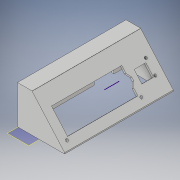
# Autodesk Inventor part: Suport - pantalla i potenciometre
Saved by Autodesk Inventor 2019 (Build 230136000, 136)
## iProperties
Created: 2018-08-18
Part Number: Suport - pantalla i potenciometre
Material: Genérico
Document SubType Name: Modeling
Designer: Albert Garangou Culebras
Density: 1 g/cm^3
Appearance: Valor por defecto
Author: Albert Garangou Culebras
Autodesk Inventor part; units mm, degrees
ref_plane "YZ Plane" through (0, 0, 0) normal (1, 0, 0) x (0, 1, 0)
ref_plane "XZ Plane" through (0, 0, 0) normal (0, 1, 0) x (-1, 0, 0)
ref_plane "XY Plane" through (0, 0, 0) normal (0, 0, 1) x (1, 0, 0)
sketch "Boceto3" plane through (0, 0, 0) normal (0, 0, 1) x (1, 0, 0)
  line L0 (40, 0) -> (37, 0)
  line L1 (0, 0) -> (0, 45)
  line L2 (0, 45) -> (3, 45)
  line L3 (40, 0) -> (40, 3)
  line L4 (40, 3) -> (3, 45)
  line L5 (0, 0) -> (40, 0)
  dimension "d3" = 3
  dimension "d4" = 45
  dimension "d5" = 3
  dimension "d6" = 3
  constraints: 12 end point, 2 horizontal, 2 vertical, 1 perpendicular
  measures "d3" distance of L0.start L0.end
  measures "d4" distance of L1.start L1.end
  measures "d5" distance of L1.end L2.end
  measures "d6" distance of L0.start L3.end
extrude "Extrusión1" add sketch "Boceto3" against normal blind 98.2
sketch "Boceto4" plane through (0, 0, 0) normal (0, 0, 1) x (1, 0, 0)
  line L0 (3.3154, 41.6201) -> (2, 43)
  line L1 (3.3154, 41.6201) -> (38, 2)
  line L2 (38, 2) -> (2, 2)
  line L3 (2, 2) -> (2, 43)
  point P0 (0, 45)
  constraints: 8 end point, 1 horizontal
extrude "Extrusión2" cut sketch "Boceto4" against normal blind 210.55
sketch "Boceto6" plane through (0, 0, 0) normal (0, 0, 1) x (1, 0, 0)
  line L0 (1.0395, 0.9992) -> (39.0395, 0.9992)
  line L1 (39.0395, 1.0003) -> (39.0395, 1.9993) projected
  line L2 (39.0395, 0.9992) -> (39.0395, 1.9993)
  line L3 (39.0395, 1.9993) -> (3, 44.0003)
  line L4 (2.88, 44.0003) -> (1, 44.0003) projected
  line L5 (3, 44.0003) -> (1, 44.0003)
  line L6 (1, 1.0003) -> (39.0395, 1.0003) projected
  line L7 (1, 44.0003) -> (1, 1.0003)
  point P0 (0, 0)
  constraints: 10 end point, 2 perpendicular, 1 horizontal, 1 parallel
extrude "Extrusión3" add sketch "Boceto6" against normal blind 2
sketch "Boceto7" plane through (0, 0, -98.2) normal (0, 0, -1) x (-1, 0, 0)
  line L0 (-1, 1.0003) -> (-39.0395, 1.0003) projected
  line L1 (-1, 1.0003) -> (-39.0395, 1.0003)
  line L2 (-39.0395, 1.0003) -> (-39.0395, 2)
  line L3 (-39.0395, 1.9993) -> (-2.88, 44.0003) projected
  line L4 (-39.0395, 2) -> (-2.88, 44.0003)
  line L5 (-2.88, 44.0003) -> (-1, 44.0003) projected
  line L6 (-1, 44.0003) -> (-1, 1.0003)
  line L7 (-2.88, 44.0003) -> (6.9067, 55.3678)
  line L8 (6.9067, 55.3678) -> (10.1689, 59.157)
  line L9 (10.1689, 59.157) -> (10.1689, 0)
  line L10 (10.1689, 0) -> (0, 0)
  dimension "d68" = 15
  dimension "d70" = 5
  constraints: 17 end point, 2 perpendicular, 2 vertical, 1 collinear
  measures "d68" distance of L3.end L7.end
  measures "d70" distance of L7.end L8.end
extrude "Extrusión4" add sketch "Boceto7" against normal blind 2
sketch "Boceto10" plane through (0, 0, -96.2) normal (0, 0, 1) x (1, 0, 0)
  line L0 (20.1691, 1.0003) -> (21.6691, 1.0003)
  line L1 (39.0395, 1.0003) -> (1, 1.0003) projected
  line L2 (21.6691, 1.0003) -> (21.6691, 22.1759)
  line L3 (2.88, 44.0003) -> (39.0395, 1.9993) projected
  line L4 (21.6691, 22.1759) -> (20.1691, 23.9182)
  line L5 (20.1691, 23.9182) -> (20.1691, 1.0003)
  point P0 (0, 0)
  dimension "d49" = 1.5
  constraints: 8 end point, 2 point on line, 1 collinear, 1 parallel, 1 vertical
  measures "d49" distance of L0.start L0.end
extrude "Extrusión7" add sketch "Boceto10" along normal blind 96
sketch "Boceto15" plane through (0, 0, -98.2) normal (0, 0, -1) x (-1, 0, 0)
  line L0 (-3, 45) -> (-40, 3) projected
  line L1 (-20.3927, 25.257) -> (-7.1721, 40.2641)
  line L2 (-7.1721, 40.2641) -> (-7.1721, 0)
  line L3 (-20.1691, 1.0003) -> (-1, 1.0003) projected
  line L4 (-7.1721, 40.2641) -> (-3, 45)
  line L5 (0, 45) -> (-3, 45)
  line L6 (0, 0) -> (0, 45) projected
  line L7 (0, 45) -> (0, 0)
  line L8 (0, 0) -> (-7.1721, 0)
  line L9 (-40, 0) -> (0, 0) projected
  dimension "d71" = 20
  constraints: 12 end point, 3 collinear, 2 point on line, 1 horizontal, 1 perpendicular
  measures "d71" distance of L1.start L1.end
extrude "Extrusión9" cut sketch "Boceto15" against normal blind 617.4
sketch "Boceto16" plane through (0, 0, -96.2) normal (0, 0, 1) x (1, 0, 0)
  line L0 (7.1721, 1) -> (8.6721, 1.0003)
  line L1 (20.1691, 1.0003) -> (7.1721, 1.0003) projected
  line L2 (8.6721, 1.0003) -> (8.6721, 37.2725)
  line L3 (7.1721, 39.0149) -> (20.1691, 23.9182) projected
  line L4 (8.6721, 37.2725) -> (7.1721, 39.0149)
  line L5 (7.1721, 39.0149) -> (7.1721, 1)
  point P0 (0, 0)
  dimension "d74" = 1.5
  constraints: 8 end point, 1 collinear, 1 parallel, 1 perpendicular, 1 point on line
  measures "d74" distance of L0.start L0.end
extrude "Extrusión10" add sketch "Boceto16" along normal blind 95.4
sketch "Boceto17" plane through (0, 0, 0) normal (0, 0, 1) x (1, 0, 0)
  line L0 (20.1691, 1.0003) -> (8.6721, 1.0003) projected
  line L1 (8.6721, 35.5011) -> (8.6721, 2) projected
  line L2 (8.6721, 1.0003) -> (8.6721, 37.2725)
  line L3 (39.0395, 1.9993) -> (21.6691, 22.1759) projected
  line L4 (8.6721, 37.2725) -> (39.0395, 1.9993)
  line L5 (39.0395, 1.9993) -> (39.0395, 1.0003)
  line L6 (39.0395, 1.0003) -> (8.6721, 1.0003)
  line L7 (40, 0) -> (7.1721, 0) projected
  point P0 (0, 0)
  constraints: 8 end point, 2 collinear, 2 parallel
extrude "Extrusión11" cut sketch "Boceto17" against normal blind 235.6
sketch "Boceto21" plane through (40, 3, 0) normal (0.750359, 0.6610305, 0) x (0, 0, -1)
  line L0 (85, 24.1901) -> (85, 18.1901)
  line L1 (76, 24.1901) -> (81, 24.1901)
  line L2 (81, 24.1901) -> (85, 24.1901)
  line L3 (77, 12.1901) -> (76, 12.1901)
  line L4 (77, 12.1901) -> (77, 11.1901)
  line L5 (5, 11.1901) -> (5, 12.1901)
  line L6 (5, 11.1901) -> (5, 7.1901)
  line L7 (5, 7.1901) -> (77, 7.1901)
  line L8 (77, 7.1901) -> (77, 11.1901)
  line L9 (77, 32.1901) -> (5, 32.1901)
  line L10 (5, 7.1901) -> (5, 32.1901)
  line L11 (77, 12.1901) -> (77, 32.1901)
  line L12 (85, 18.1901) -> (85, 13.1901)
  line L13 (98.2, 19.2082) -> (98.2, -0.8655) projected
  line L14 (97, 18.1901) -> (97, 13.1901)
  line L15 (85, 13.1901) -> (97, 13.1901)
  line L16 (85, 25.1901) -> (97, 25.1901)
  line L17 (85, 24.1901) -> (85, 25.1901)
  line L18 (97, 25.1901) -> (97, 18.1901)
  line L19 (0, 19.2082) -> (98.2, 19.2082) projected
  point P0 (0, 24.1901)
  dimension "d114" = 5
  dimension "d177" = 1
  dimension "d184" = 4
  dimension "d186" = 5
  constraints: 36 end point, 4 vertical, 3 horizontal, 2 perpendicular, 1 point on line
  measures "d114" distance of L1.end L1.start
  measures "d177" distance of L3.start L4.end
  measures "d184" distance of L5.start L6.end
  measures "d186" distance of L0.end L12.end
extrude "Extrusión13" cut sketch "Boceto21" against normal blind 1.5 contours L17 L16 L18 L19 L0 | L19 L18 L14 L15 L12 L0 | L19 L10 L9 L11 | L11 L4 L8 L7 L6 L5 L10 L19
sketch "Boceto22" plane through (0, 0, 0) normal (0, 0, 1) x (1, 0, 0)
  line L0 (8.6721, 1.0003) -> (39.0395, 1.0003) projected
  line L1 (8.6721, 1.0003) -> (39.0395, 1.0003)
  line L2 (39.0395, 1.0003) -> (39.0395, 2)
  line L3 (39.0395, 2) -> (8.6721, 37)
  line L4 (8.6721, 37.2725) -> (8.6721, 1.0003) projected
  line L5 (8.6721, 37) -> (8.6721, 1.0003)
  line L6 (7.1721, 0) -> (7.1721, 40.2641) projected
  line L7 (7.1721, 40.2641) -> (7.1721, 0)
  line L8 (40, 3) -> (40, 0) projected
  line L9 (7.1721, 0) -> (40, 0)
  line L10 (40, 0) -> (40, 3)
  line L11 (40, 3) -> (7.1721, 40.2641)
  line L12 (7.1721, 40.2641) -> (40, 3) projected
  point P0 (0, 0)
  constraints: 16 end point, 3 collinear, 3 perpendicular, 1 horizontal
extrude "Extrusión14" add sketch "Boceto22" along normal blind 2
sketch "Boceto24" plane through (0, 0, 2) normal (0, 0, 1) x (1, 0, 0)
  line L0 (8.6721, 1.0003) -> (8.6721, 37) projected
  line L1 (39.0395, 1.0003) -> (8.6721, 1.0003) projected
  line L2 (8.6721, 1.0003) -> (39.0395, 1.0003)
  line L3 (39.0395, 1.0003) -> (39.0395, 2)
  line L4 (39.0395, 2) -> (8.6721, 37)
  line L5 (8.6721, 37) -> (8.6721, 1.0003)
  point P0 (0, 0)
  constraints: 8 end point, 1 collinear, 1 parallel, 1 perpendicular
extrude "Extrusión15" add sketch "Boceto24" against normal blind 2
sketch "Boceto25" plane through (0, 0, -98.2) normal (0, 0, -1) x (-1, 0, 0)
  line L0 (-8.6721, 1.0003) -> (-8.6721, 37.2725) projected
  line L1 (-8.6721, 1.0003) -> (-8.6721, 37.2725)
  line L2 (-8.6721, 37.2725) -> (-39, 2)
  line L3 (-39, 2) -> (-39, 1.0003)
  line L4 (-39, 1.0003) -> (-8.6721, 1.0003)
  line L5 (-7.1721, 0) -> (-40, 0) projected
  line L6 (-7.1721, 40) -> (-7.1721, 0)
  line L7 (-40, 0) -> (-7.1721, 0)
  line L8 (-40, 0) -> (-40, 2.8598)
  line L9 (-7.1721, 0) -> (-7.1721, 40.2641) projected
  line L10 (-40, 2.8598) -> (-7.1721, 40.2641)
  point P0 (0, 0)
  constraints: 16 end point, 2 parallel, 2 vertical, 1 collinear, 1 perpendicular
extrude "Extrusión16" add sketch "Boceto25" along normal blind 7
sketch "Boceto27" plane through (0, 0, -105.2) normal (0, 0, -1) x (-1, 0, 0)
  line L0 (-8.6721, 1.0003) -> (-39.0395, 1.0003) projected
  line L1 (-8.6721, 1.0003) -> (-39.0395, 1.0003)
  line L2 (-39.0395, 1.0003) -> (-39.0395, 1.9993)
  line L3 (-8.6721, 1.0003) -> (-8.6721, 37.2725) projected
  line L4 (-39.0395, 1.9993) -> (-8.6721, 37.2725)
  line L5 (-8.6721, 37.2725) -> (-8.6721, 1.0003)
  point P0 (0, 0)
  constraints: 8 end point, 2 collinear, 1 perpendicular
extrude "Extrusión17" add sketch "Boceto27" against normal blind 2
sketch "Boceto28" plane through (7.1721, 0, 2) normal (0, -1, 0) x (1, 0, 0)
  line L0 (0, 0) -> (0, -107.2) projected
  line L1 (32.8279, 0) -> (32.8279, -107.2) projected
  line L2 (0, 0) -> (32.8279, 0)
  line L3 (32.8279, 0) -> (32.8279, -107.2)
  line L4 (32.8279, -107.2) -> (0, -107.2)
  line L5 (0, -107.2) -> (0, 0)
  point P0 (-7.1721, -2)
  constraints: 8 end point, 2 parallel, 1 horizontal, 1 perpendicular
extrude "Extrusión18" add sketch "Boceto28" along normal blind 2
sketch "Boceto29" plane through (7.1721, 40.2641, -98.2) normal (-1, 0, 0) x (0, 0, 1)
  line L0 (0, 0) -> (-7, 0) projected
  line L1 (100.2, -37.2641) -> (100.2, -42.2641) projected
  line L2 (-7, 0) -> (100.2, 0)
  line L3 (100.2, 0) -> (100.2, -42.2641)
  line L4 (100.2, -42.2641) -> (-7, -42.2641)
  line L5 (-7, -42.2641) -> (-7, 0)
  point P0 (98.2, -40.2641)
  constraints: 8 end point, 2 parallel, 1 horizontal, 1 perpendicular
extrude "Extrusión19" add sketch "Boceto29" along normal blind 2
sketch "Boceto30" plane through (0, 0, -105.2) normal (0, 0, -1) x (-1, 0, 0)
  line L0 (-7.1721, 40.2641) -> (-5.1721, 40.2641)
  line L1 (-5.1721, 40.2641) -> (-5.1721, -2) projected
  line L2 (-5.1721, 40.2641) -> (-5.1721, -2)
  line L3 (-40, -2) -> (-5.1721, -2) projected
  line L4 (-5.1721, -2) -> (-40, -2)
  line L5 (-40, 2.8598) -> (-40, -2) projected
  line L6 (-40, -2) -> (-40, 2.8598)
  line L7 (-40, 2.8598) -> (-7.1721, 40.2641)
  line L8 (-7.1721, 40.2641) -> (-5.1721, 40.2641)
  point P0 (0, 0)
  constraints: 12 end point, 3 collinear, 1 horizontal, 1 perpendicular
extrude "Extrusión20" add sketch "Boceto30" along normal blind 2
sketch "Boceto31" plane through (0, 0, 2) normal (0, 0, 1) x (1, 0, 0)
  line L0 (5.1721, -2) -> (5.1721, 40.2641) projected
  line L1 (5.1721, 40.2643) -> (5.1721, -2)
  line L2 (40, -2) -> (5.1721, -2) projected
  line L3 (5.1721, -2) -> (40, -2)
  line L4 (40, 2.8598) -> (40, -2) projected
  line L5 (40, -2) -> (40, 2.8598)
  line L6 (40, 2.8598) -> (7.1721, 40.2641) projected
  line L7 (7.1721, 40.2641) -> (40, 2.8598)
  line L8 (7.1721, 40.2641) -> (5.1721, 40.2641)
  point P0 (0, 0)
  constraints: 11 end point, 3 collinear, 1 horizontal
extrude "Extrusión21" add sketch "Boceto31" along normal blind 2
sketch "Boceto32" plane through (40, 3, 2) normal (0.750359, 0.6610305, 0) x (0, 0, -1)
  line L0 (-2, 49.6617) -> (-2, 0)
  line L1 (-2, 0) -> (109.2, 0)
  line L2 (109.2, -3.7518) -> (109.2, 19.2705) projected
  line L3 (100.2, -0.1052) -> (109.2, -0.1052) projected
  line L4 (109.2, 49.6617) -> (109.2, -0.1052)
  line L5 (109.2, 49.6617) -> (-2, 49.6617)
  line L6 (-2, 50.9838) -> (-2, 19.2705) projected
  line L7 (7, 11.1901) -> (7, 36.1901) projected
  line L8 (7, 36.1901) -> (7, 12.1901)
  line L9 (78, 36.1901) -> (7, 36.1901)
  line L10 (87, 13.1901) -> (87, 25.1901) projected
  line L11 (100.2, 49.6617) -> (109.2, 49.6617) projected
  line L12 (109.2, 49.6617) -> (109.2, -0.1052)
  line L13 (-2, -3.7518) -> (-2, -0.1052) projected
  line L14 (109.2, -0.1052) -> (-2, -0.1052)
  line L15 (-2, -0.1052) -> (-2, 49.6617)
  line L16 (109.2, 49.6617) -> (-2, 49.6617)
  line L17 (7, 12.1901) -> (7, 11.1901)
  line L18 (7, 11.1901) -> (79, 11.1901)
  line L19 (79, 11.1901) -> (79, 36.1901)
  line L20 (79, 36.1901) -> (78, 36.1901)
  line L21 (99, 13.1901) -> (87, 13.1901) projected
  line L22 (99, 13.1901) -> (87, 13.1901)
  line L23 (87, 13.1901) -> (87, 25.1901)
  line L24 (99, 25.1901) -> (87, 25.1901) projected
  line L25 (99, 25.1901) -> (87, 25.1901)
  line L26 (99, 25.1901) -> (99, 13.1901)
  line L27 (100.2, 46.4254) -> (100.2, -0.0893) projected
  point P0 (2, 24.1901)
  point P1 (87, 30.1901)
  point P2 (99, 30.1901)
  point P3 (87, 18.1901)
  point P4 (99, 18.1901)
  dimension "d174" = 1
  dimension "d175" = 72
  constraints: 36 end point, 6 collinear, 5 perpendicular, 2 point on line, 2 vertical, 1 horizontal, 1 parallel
  measures "d174" distance of L8.end L7.start
  measures "d175" distance of L7.start L18.end
extrude "Extrusión22" [suppressed]
sketch "Boceto33" plane through (40.7504, 3.661, 2) normal (0.750359, 0.6610305, 0) x (0, 0, -1)
  line L0 (87, 25.1901) -> (87, 13.1901) projected
  line L1 (87, 30.1901) -> (99, 30.1901) projected
  line L2 (87, 30.1901) -> (99, 30.1901)
  line L3 (99, 30.1901) -> (99, 18.1338)
  line L4 (100.2, -0.1052) -> (100.2, 49.6617) projected
  line L5 (99, 18.1338) -> (87, 18.1338)
  line L6 (87, 30.1901) -> (87, 34.1901)
  line L7 (87, 34.1901) -> (83, 34.1901)
  line L8 (99, 18.1901) -> (99, 14.1901)
  line L9 (99, 14.1901) -> (103, 14.1901)
  line L10 (83, 34.1901) -> (103, 34.1901)
  line L11 (103, 34.1901) -> (103, 14.1901)
  line L12 (103, 14.1901) -> (83, 14.1901)
  line L13 (83, 14.1901) -> (83, 34.1901)
  point P0 (2, 24.1901)
  point P1 (87, 18.1901)
  dimension "d126" = 4
  dimension "d127" = 4
  dimension "d129" = 4
  dimension "d130" = 4
  constraints: 22 end point, 4 perpendicular, 3 parallel, 2 horizontal, 2 vertical
  measures "d126" distance of L1.start L6.end
  measures "d127" distance of L6.end L7.end
  measures "d129" distance of L8.start L8.end
  measures "d130" distance of L8.end L9.end
extrude "Extrusión23" [suppressed]
sketch "Boceto34" plane through (40.7504, 3.661, 2) normal (0.750359, 0.6610305, 0) x (0, 0, -1)
  line L0 (99, 18.1901) -> (99, 30.1901)
  line L1 (99, 18.1901) -> (87, 18.1901)
  line L2 (87, 18.1901) -> (87, 30.1901)
  line L3 (99, 30.1901) -> (99, 18.1901)
  line L4 (99, 30.1901) -> (99, 18.1901)
  line L5 (87, 18.1901) -> (99, 18.1901)
  line L6 (99, 30.1901) -> (99, 31.1901)
  line L7 (99, 31.1901) -> (87, 31.1901)
  line L8 (87, 31.1901) -> (87, 30.1901)
  point P0 (2, 24.1901)
  point P1 (83, 34.1901)
  dimension "d173" = 1
  constraints: 18 end point, 3 perpendicular, 1 collinear, 1 point on line
  measures "d173" distance of L0.end L6.end
extrude "Extrusión24" [suppressed]
sketch "Boceto35" plane through (40.0695, 2.9211, 4) normal (0, 0, 1) x (0.750359, 0.6610305, 0)
  line L0 (0, 49.7669) -> (1, 49.7669) projected
  line L1 (1, 49.7669) -> (0, 49.7669)
  line L2 (0, 49.7669) -> (0, 0)
  line L3 (0, 0) -> (1, 0) projected
  line L4 (0, 0) -> (1, 0)
  line L5 (1, 0) -> (1, 49.7669)
  point P0 (-31.9975, 24.2953)
  constraints: 8 end point, 3 perpendicular, 1 horizontal
extrude "Extrusión25" [suppressed]
sketch "Boceto36" plane through (0, 0, 4) normal (0, 0, 1) x (1, 0, 0)
  line L0 (5.1721, 40.2641) -> (7.1721, 40.2641) projected
  line L1 (7.1721, 40.2641) -> (40, 2.8598) projected
  line L2 (5.1721, 40.2641) -> (7.1721, 40.2641)
  line L3 (7.1721, 40.2641) -> (7.9224, 40.9252) projected
  line L4 (7.1721, 40.2641) -> (7.9224, 40.9252)
  line L5 (7.9224, 40.9252) -> (6.6004, 42.4259)
  line L6 (6.6004, 42.4259) -> (5.1721, 42.4259)
  line L7 (5.1721, -2) -> (5.1721, 40.2641) projected
  line L8 (5.1721, 42.4259) -> (5.1721, 40.2641)
  point P0 (0, 0)
  dimension "d140" = 2
  constraints: 10 end point, 2 perpendicular, 1 collinear, 1 horizontal, 1 parallel
  measures "d140" distance of L3.end L5.end
extrude "Extrusión26" add sketch "Boceto36" against normal blind 111.22
sketch "Boceto37" plane through (0, 0, 4) normal (0, 0, 1) x (1, 0, 0)
  line L0 (40.0695, 2.9211) -> (7.1721, 40.2641) projected
  line L1 (40.0695, 2.9211) -> (39.9946, 2.8551)
  line L2 (39.9946, 2.8551) -> (7.1346, 40.2311)
  line L3 (7.1721, 40.2641) -> (7.9224, 40.9252) projected
  line L4 (7.1346, 40.2311) -> (7.9224, 40.9252)
  line L5 (7.9224, 40.9252) -> (40.0695, 2.9211)
  point P0 (0, 0)
  constraints: 8 end point, 1 collinear, 1 perpendicular
extrude "Extrusión27" add sketch "Boceto37" against normal blind 2 contours L1 L2 L4 L0
sketch "Boceto38" plane through (0, 0, 4) normal (0, 0, 1) x (1, 0, 0)
  line L0 (40, 2.8598) -> (40, -2) projected
  line L1 (40, -2) -> (40, 2.8598)
  line L2 (40.0695, 2.9211) -> (40.8199, 3.5821) projected
  line L3 (40, 2.8598) -> (40.8199, 3.5821)
  line L4 (40, -2) -> (42, -2)
  line L5 (42, -2) -> (42, 2.2425)
  line L6 (42, 2.2425) -> (40.8199, 3.5821)
  point P0 (0, 0)
  constraints: 10 end point, 2 collinear, 1 perpendicular
extrude "Extrusión28" add sketch "Boceto38" against normal blind 111.25
sketch "Boceto39" plane through (0, 0, -107.2) normal (0, 0, -1) x (-1, 0, 0)
  line L0 (-40.0695, 2.9211) -> (-40.8199, 3.5821) projected
  line L1 (-40.0695, 2.9211) -> (-40, 2.8598)
  line L2 (-40.0695, 2.9211) -> (-7.1721, 40.2641) projected
  line L3 (-40, 2.8598) -> (-7.1721, 40.2641)
  line L4 (-7.1721, 40.2641) -> (-40.0695, 2.9211)
  line L5 (-40.0695, 2.9211) -> (-40, 2.8598)
  point P0 (0, 0)
  constraints: 8 end point, 2 collinear, 1 perpendicular
extrude "Extrusión29" add sketch "Boceto39" against normal blind 2
sketch "Boceto40" plane through (7.1721, -2, 2) normal (0, -1, 0) x (1, 0, 0)
  line L0 (7.7868, -16.0487) -> (16.7678, -16.0487) construction
  line L1 (16.7678, -16.0487) -> (16.7678, -19.0967) construction
  line L2 (16.7678, -19.0967) -> (7.7868, -19.0967) construction
  line L3 (7.7868, -19.0967) -> (7.7868, -16.0487) construction
  spline S0 degree 2 poles (12.5423, -20.2752) (12.5423, -20.73) (12.1962, -21.427) (11.9095, -21.6544) knots 0 0 0 1 2 2 2
  spline S1 degree 2 poles (11.9095, -21.6544) (11.5635, -21.9213) (10.7775, -22.1487) (10.1547, -22.1487) knots 0 0 0 1 2 2 2
  line L4 (10.1547, -22.1487) -> (8.4047, -22.1487)
  line L5 (8.4047, -22.1487) -> (8.4047, -16.0487)
  line L6 (8.4047, -16.0487) -> (10.0212, -16.0487)
  spline S2 degree 2 poles (10.0212, -16.0487) (10.6737, -16.0487) (11.3262, -16.1327) (11.6228, -16.2959) knots 0 0 0 1 2 2 2
  spline S3 degree 2 poles (11.6228, -16.2959) (11.954, -16.4689) (12.2556, -17.0374) (12.2556, -17.4229) knots 0 0 0 1 2 2 2
  spline S4 degree 2 poles (12.2556, -17.4229) (12.2556, -17.853) (11.8008, -18.5352) (11.4004, -18.728) knots 0 0 0 1 2 2 2
  line L7 (11.4004, -18.728) -> (11.4004, -18.7576)
  spline S5 degree 2 poles (11.4004, -18.7576) (11.9441, -18.9059) (12.5423, -19.6919) (12.5423, -20.2752) knots 0 0 0 1 2 2 2
  spline S6 degree 2 poles (11.697, -20.3098) (11.697, -19.9638) (11.4992, -19.5189) (11.2026, -19.3607) knots 0 0 0 1 2 2 2
  spline S7 degree 2 poles (11.2026, -19.3607) (11.0099, -19.2618) (10.5551, -19.2025) (10.1349, -19.2025) knots 0 0 0 1 2 2 2
  line L8 (10.1349, -19.2025) -> (9.2154, -19.2025)
  line L9 (9.2154, -19.2025) -> (9.2154, -21.4566)
  line L10 (9.2154, -21.4566) -> (9.8729, -21.4566)
  spline S8 degree 2 poles (9.8729, -21.4566) (10.4068, -21.4566) (11.0197, -21.3578) (11.257, -21.1996) knots 0 0 0 1 2 2 2
  spline S9 degree 2 poles (11.257, -21.1996) (11.4844, -21.0365) (11.697, -20.6311) (11.697, -20.3098) knots 0 0 0 1 2 2 2
  spline S10 degree 2 poles (11.4103, -17.5366) (11.4103, -17.3191) (11.262, -16.9929) (11.0988, -16.8989) knots 0 0 0 1 2 2 2
  spline S11 degree 2 poles (11.0988, -16.8989) (10.9011, -16.7902) (10.4216, -16.7408) (9.9915, -16.7408) knots 0 0 0 1 2 2 2
  line L11 (9.9915, -16.7408) -> (9.2154, -16.7408)
  line L12 (9.2154, -16.7408) -> (9.2154, -18.5253)
  line L13 (9.2154, -18.5253) -> (10.1349, -18.5253)
  spline S12 degree 2 poles (10.1349, -18.5253) (10.5155, -18.5253) (10.8764, -18.4462) (11.0692, -18.3226) knots 0 0 0 1 2 2 2
  spline S13 degree 2 poles (11.0692, -18.3226) (11.257, -18.204) (11.4103, -17.8233) (11.4103, -17.5366) knots 0 0 0 1 2 2 2
  line L14 (12.6906, -22.1487) -> (14.747, -16.0487)
  line L15 (14.747, -16.0487) -> (15.7455, -16.0487)
  line L16 (15.7455, -16.0487) -> (17.8019, -22.1487)
  line L17 (17.8019, -22.1487) -> (16.9467, -22.1487)
  line L18 (16.9467, -22.1487) -> (16.3931, -20.4433)
  line L19 (16.3931, -20.4433) -> (14.0648, -20.4433)
  line L20 (14.0648, -20.4433) -> (13.5111, -22.1487)
  line L21 (13.5111, -22.1487) -> (12.6906, -22.1487)
  line L22 (16.1706, -19.7512) -> (15.2265, -16.8792)
  line L23 (15.2265, -16.8792) -> (14.2872, -19.7512)
  line L24 (14.2872, -19.7512) -> (16.1706, -19.7512)
  line L25 (20.5059, -22.1487) -> (18.143, -22.1487)
  line L26 (18.143, -22.1487) -> (18.143, -21.5258)
  line L27 (18.143, -21.5258) -> (18.9191, -21.5258)
  line L28 (18.9191, -21.5258) -> (18.9191, -16.6716)
  line L29 (18.9191, -16.6716) -> (18.143, -16.6716)
  line L30 (18.143, -16.6716) -> (18.143, -16.0487)
  line L31 (18.143, -16.0487) -> (20.5059, -16.0487)
  line L32 (20.5059, -16.0487) -> (20.5059, -16.6716)
  line L33 (20.5059, -16.6716) -> (19.7298, -16.6716)
  line L34 (19.7298, -16.6716) -> (19.7298, -21.5258)
  line L35 (19.7298, -21.5258) -> (20.5059, -21.5258)
  line L36 (20.5059, -21.5258) -> (20.5059, -22.1487)
  line L37 (25.726, -22.1487) -> (24.7966, -22.1487)
  line L38 (24.7966, -22.1487) -> (23.3137, -19.7166)
  line L39 (23.3137, -19.7166) -> (21.801, -22.1487)
  line L40 (21.801, -22.1487) -> (20.9261, -22.1487)
  line L41 (20.9261, -22.1487) -> (22.8688, -19.0938)
  line L42 (22.8688, -19.0938) -> (20.9854, -16.0487)
  line L43 (20.9854, -16.0487) -> (21.9147, -16.0487)
  line L44 (21.9147, -16.0487) -> (23.368, -18.4363)
  line L45 (23.368, -18.4363) -> (24.851, -16.0487)
  line L46 (24.851, -16.0487) -> (25.726, -16.0487)
  line L47 (25.726, -16.0487) -> (23.8179, -19.0542)
  line L48 (23.8179, -19.0542) -> (25.726, -22.1487)
  point P0 (-7.1721, -2)
  constraints: 2 other
extrude "Extrusión30" cut sketch "Boceto40" against normal blind 0.5
sketch "Boceto41" plane through (8.6721, 1.0003, 0) normal (0, 1, 0) x (1, 0, 0)
  circle A0 centre (15, 56) radius 1.6
  circle A1 centre (15, 23) radius 1.6
  point P0 (-8.6721, 0)
  dimension "d68" = 15
  dimension "d155" = 3.2
  dimension "d156" = 3.2
  constraints: 2 centre point
  measures "d155" diameter of A0
  measures "d156" diameter of A1
extrude "Extrusión31" cut sketch "Boceto41" against normal blind 65.25
sketch "Boceto42" plane through (5.1721, 40.2641, -98.2) normal (-1, 0, 0) x (0, 0, 1)
  line L0 (9.7, -39.2638) -> (9.7, -34.2638)
  line L1 (9.7, -34.2638) -> (24.7, -34.2638)
  line L2 (24.7, -34.2638) -> (24.7, -39.2638)
  line L3 (9.7, -39.2638) -> (24.7, -39.2638)
  line L4 (0, -39.2638) -> (98.2, -39.2638) projected
  point P0 (98.2, -40.2641)
  point P1 (17.2, -27.608)
  constraints: 8 end point, 2 perpendicular, 1 collinear
extrude "Extrusión32" cut sketch "Boceto42" against normal blind 6.25
sketch "Boceto43" plane through (5.1721, 40.2641, -98.2) normal (-1, 0, 0) x (0, 0, 1)
  line L0 (21.2, -10.7488) -> (93.2, -10.7488) projected
  line L1 (93.2, -10.7488) -> (40, -10.7488)
  line L2 (40, -10.7488) -> (40, -15.7488)
  line L3 (40, -15.7488) -> (93.2, -15.7488)
  line L4 (93.2, -15.7488) -> (93.2, -10.7488)
  line L5 (93.2, -35) -> (40, -35)
  line L6 (40, -35) -> (40, -30)
  line L7 (40, -30) -> (93.2, -30)
  line L8 (93.2, -30) -> (93.2, -35)
  line L9 (103, -15.7488) -> (118.5563, -15.7488) construction
  point P0 (98.2, -40.2641)
  point P1 (22.2, -10.7488)
  dimension "d164" = 5
  dimension "d165" = 5
  constraints: 18 end point, 4 parallel, 3 horizontal, 2 perpendicular
  measures "d164" distance of L2.end L1.end
  measures "d165" distance of L5.end L6.end
sketch "Boceto44" plane through (0, 0, 4) normal (0, 0, 1) x (1, 0, 0)
  line L0 (5.1721, -2) -> (5.1721, 40.2641) projected
  line L1 (5.1721, 19.1321) -> (16, 6.2278)
  line L2 (5.1721, 19.1321) -> (22.0173, 19.1321) construction
  point P0 (0, 0)
  dimension "d167" = 50
  constraints: 4 end point, 1 equal length, 1 horizontal, 1 midpoint
  measures "d167" angle of L1 L2
sweep "Barrido1" cut profiles "Boceto43" path "Boceto44" path curves L1
sketch "Boceto45" plane through (7.1721, -2, 2) normal (0, -1, 0) x (1, 0, 0)
  line L0 (4.0953, -60.2) -> (8.2908, -60.2)
  line L1 (8.2908, -7) -> (4.0953, -7)
  line L2 (8.2908, -7) -> (0, -7)
  line L3 (0, -7) -> (0, -60.2)
  line L4 (0, -60.2) -> (8.2908, -60.2)
  line L5 (8.2908, -60.2) -> (8.2908, -7)
  point P0 (-7.1721, -2)
  constraints: 12 end point, 3 parallel, 2 horizontal, 1 perpendicular
extrude "Extrusión33" add sketch "Boceto45" against normal blind 3
sketch "Boceto46" plane through (8.6721, 1.0003, 0) normal (0, 1, 0) x (1, 0, 0)
  line L0 (-3.5, 73.5) -> (-3.5, 88.5) projected
  line L1 (-3.5, 73.5) -> (-3.5, 88.5)
  point P0 (-8.6721, 0)
  constraints: 2 end point, 1 collinear
ref_plane "Plano de trabajo5" through (5.1721, 1.0003, 4) normal (0, -1, 0) x (1, 0, 0)
sketch "Boceto47" plane through (5.1721, 1.0003, 4) normal (0, -1, 0) x (1, 0, 0)
  line L0 (36.8279, 0) -> (36.8279, -111.25) projected
  line L1 (0, 0) -> (0, -111.22) projected
  line L2 (36.8279, -111.25) -> (0, -111.25)
  line L3 (0, -111.25) -> (0, 0)
  line L4 (0, 0) -> (36.8279, 0)
  line L5 (36.8279, 0) -> (36.8279, -111.25)
  point P0 (-5.1721, -4)
  constraints: 8 end point, 2 parallel, 1 horizontal, 1 perpendicular
extrude "Extrusión34" cut sketch "Boceto47" along normal blind 22.5
sketch "Boceto48" plane through (5.1721, 40.2641, -98.2) normal (-1, 0, 0) x (0, 0, 1)
  line L0 (-9.02, 2.1617) -> (-9.02, 0.661) projected
  line L1 (102.2, -39.2638) -> (-9.05, -39.2638) projected
  line L2 (-9.02, 2.1617) -> (102.2, 2.1617)
  line L3 (102.2, 2.1617) -> (102.2, -39.2638)
  line L4 (102.2, -39.2638) -> (-9.02, -39.2638)
  line L5 (-9.02, -39.2638) -> (-9.02, 2.1617)
  point P0 (98.2, -40.2641)
  constraints: 8 end point, 2 parallel, 1 horizontal, 1 perpendicular
extrude "Extrusión35" cut sketch "Boceto48" against normal blind 3.5
sketch "Boceto49" plane through (8.6721, 40.2641, -98.2) normal (-1, 0, 0) x (0, 0, 1)
  line L0 (-9, -39.2638) -> (-5, -39.2638)
  line L1 (-5, -39.2638) -> (-5, -2.9916) projected
  line L2 (-5, -39.2638) -> (-5, -2.9916)
  line L3 (98.2, -39.2638) -> (98.2, -2.9916) projected
  line L4 (-5, -2.9916) -> (98.2, -2.9916)
  line L5 (98.2, -2.9916) -> (98.2, -39.2638)
  line L6 (102.2, -39.2638) -> (98.2, -39.2638) projected
  line L7 (98.2, -39.2638) -> (102.2, -39.2638)
  line L8 (102.2, -39.2638) -> (102.2, 0)
  line L9 (102.2, 0) -> (-9, 0)
  line L10 (0, -1.7027) -> (-7, -1.7027) projected
  line L11 (-5, -39.2638) -> (-9, -39.2638) projected
  line L12 (-9, 0) -> (-9, -39.2638)
  point P0 (98.2, -40.2641)
  constraints: 16 end point, 5 perpendicular, 1 collinear, 1 horizontal, 1 parallel
extrude "Extrusión36" add sketch "Boceto49" along normal blind 15
sketch "Boceto50" plane through (40, 3, 2) normal (0.750359, 0.6610305, 0) x (0, 0, -1)
  line L0 (-2, -0.1052) -> (0, -0.1052) projected
  line L1 (109.2, 47.3926) -> (107.2, 47.3926) projected
  line L2 (-2, -0.1052) -> (109.2, -0.1052)
  line L3 (109.2, -0.1052) -> (109.2, 47.3926)
  line L4 (109.2, 47.3926) -> (-2, 47.3926)
  line L5 (-2, 47.3926) -> (-2, -0.1052)
  line L6 (87, 25.1901) -> (87, 13.1901) projected
  line L7 (87, 25.1901) -> (99, 25.1901)
  line L8 (99, 25.1901) -> (99, 13.1901) projected
  line L9 (99, 25.1901) -> (99, 13.1901)
  line L10 (99, 13.1901) -> (87, 13.1901)
  line L11 (79, 7.1901) -> (79, 32.1901)
  line L12 (79, 32.1901) -> (7, 32.1901) projected
  line L13 (79, 32.1901) -> (7, 32.1901)
  line L14 (7, 7.1901) -> (7, 32.1901) projected
  line L15 (7, 32.1901) -> (7, 7.1901)
  line L16 (79, 7.1901) -> (79, 32.1901) projected
  line L17 (7, 7.1901) -> (79, 7.1901)
  line L18 (99, 13.1901) -> (99, 25.1901) projected
  line L19 (87, 13.1901) -> (99, 13.1901)
  line L20 (99, 13.1901) -> (99, 25.1901)
  line L21 (99, 25.1901) -> (87, 25.1901)
  line L22 (87, 25.1901) -> (87, 13.1901)
  point P0 (2, 24.1901)
  constraints: 30 end point, 6 equal length, 5 perpendicular, 3 horizontal, 1 vertical
extrude "Extrusión37" add sketch "Boceto50" along normal blind 1 contours L5 L4 L1 L3 L2 L0 | L7 L8 L10 L6
sketch "Boceto51" plane through (42, 2.2425, 4) normal (0.750359, 0.6610305, 0) x (0, 0, -1)
  line L0 (89, 15.0806) -> (101, 15.0806) projected
  line L1 (89, 15.0806) -> (101, 15.0806)
  line L2 (89, 27.0806) -> (89, 15.0806) projected
  line L3 (89, 15.0806) -> (89, 27.0806)
  line L4 (101, 27.0806) -> (89, 27.0806) projected
  line L5 (89, 27.0806) -> (101, 27.0806)
  line L6 (101, 15.0806) -> (101, 27.0806) projected
  line L7 (101, 27.0806) -> (101, 15.0806)
  point P0 (4, 26.0806)
  constraints: 8 end point, 4 collinear
extrude "Extrusión38" cut sketch "Boceto51" against normal blind 79.5
sketch "Boceto52" plane through (0, 0, -103.2) normal (0, 0, 1) x (1, 0, 0)
  line L0 (-6.3279, 40.2641) -> (-6.3279, 1.0003) projected
  line L1 (-6.3279, 1.0003) -> (-6.3279, 37.2725)
  line L2 (8.6721, 37.2725) -> (-6.3279, 37.2725) projected
  line L3 (-6.3279, 1.0003) -> (-6.3279, 37.2725) projected
  line L4 (-6.3279, 37.2725) -> (-3.8279, 37.2725)
  line L5 (-3.8279, 37.2725) -> (-3.8279, 1.0003)
  line L6 (39, 1.0003) -> (-6.3279, 1.0003) projected
  line L7 (-6.3279, 1.0003) -> (-3.8279, 1.0003)
  point P0 (0, 0)
  dimension "d193" = 2.5
  constraints: 8 end point, 2 point on line, 1 collinear, 1 perpendicular, 1 vertical
  measures "d193" distance of L1.end L4.end
extrude "Extrusión39" add sketch "Boceto52" along normal blind 105.75
sketch "Boceto53" plane through (0, 0, 4) normal (0, 0, 1) x (1, 0, 0)
  line L0 (8.6721, 38.5614) -> (9.4224, 39.2225) projected
  line L1 (9.4224, 39.2225) -> (8.6233, 40.1295)
  line L2 (8.6233, 40.1295) -> (8.6233, 38.2787)
  line L3 (8.6721, 38.5614) -> (8.6721, 40.2641) projected
  line L4 (8.6233, 38.2787) -> (9.4224, 39.2225)
  point P0 (0, 0)
  constraints: 6 end point, 1 parallel, 1 perpendicular
extrude "Extrusión40" add sketch "Boceto53" against normal blind 111.2
sketch "Boceto54" plane through (-6.3279, 40.2641, -98.2) normal (-1, 0, 0) x (0, 0, 1)
  line L0 (-9, -39.2638) -> (6, -39.2638)
  line L1 (-9, -39.2638) -> (102.2, -39.2638) projected
  line L2 (6, -39.2638) -> (6, -34.2638)
  line L3 (-5, -39.2638) -> (98.2, -39.2638) projected
  line L4 (21, -39.2638) -> (6, -39.2638)
  line L5 (6, -34.2638) -> (6, -35.7638)
  line L6 (6, -35.7638) -> (21, -35.7638)
  line L7 (21, -35.7638) -> (26, -35.7638)
  line L8 (26, -35.7638) -> (26, -39.2638)
  line L9 (26, -39.2638) -> (21, -39.2638)
  point P0 (98.2, -40.2641)
  point P1 (6, -39)
  point P2 (21, -39)
  dimension "d198" = 15
  dimension "d199" = 5
  dimension "d224" = 1.5
  dimension "d225" = 5
  constraints: 16 end point, 5 point on line, 3 perpendicular, 2 collinear, 1 horizontal
  measures "d198" distance of L0.start L0.end
  measures "d199" distance of L0.end L2.end
  measures "d224" distance of L2.end L5.end
  measures "d225" distance of L6.end L7.end
extrude "Extrusión41" cut sketch "Boceto54" against normal blind 4
sketch "Boceto55" plane through (-6.3279, 40.2641, -98.2) normal (-1, 0, 0) x (0, 0, 1)
  line L0 (102.2, 0) -> (-9, 0) projected
  line L1 (98.2, -38.2648) -> (0, -38.2648) projected
  line L2 (98.2, -16) -> (43.2, -16)
  line L3 (43.2, -16) -> (43.2, -11)
  line L4 (43.2, -11) -> (98.2, -11)
  line L5 (98.2, -11) -> (98.2, -16)
  line L6 (98.2, -24) -> (43.2, -24)
  line L7 (43.2, -24) -> (43.2, -29)
  line L8 (43.2, -29) -> (98.2, -29)
  line L9 (98.2, -24) -> (98.2, -29)
  point P0 (98.2, -40.2641)
  constraints: 16 end point, 2 perpendicular
sketch "Boceto56" plane through (0, 0, 4) normal (0, 0, 1) x (1, 0, 0)
  line L0 (-6, 23) -> (1.5519, 14)
  line L1 (-6, 23) -> (5.7487, 23) construction
  point P0 (0, 0)
  dimension "d205" = 50
  constraints: 4 end point, 1 equal length, 1 horizontal
  measures "d205" angle of L0 L1
sweep "Barrido2" cut profiles "Boceto55" path "Boceto56"
sketch "Boceto57" plane through (-6.3279, 40.2641, -98.2) normal (-1, 0, 0) x (0, 0, 1)
  circle A0 centre (38, -11) radius 2.45
  point P0 (98.2, -40.2641)
  dimension "d211" = 4.9
  constraints: 1 centre point
  measures "d211" diameter of A0
extrude "Extrusión42" cut sketch "Boceto57" against normal blind 5
sketch "Boceto59" plane through (42, 2.2425, 4) normal (0.750359, 0.6610305, 0) x (0, 0, -1)
  line L0 (9, 34.0806) -> (9, 9.0806) projected
  line L1 (81, 9.0806) -> (81, 34.0806) projected
  line L2 (81, 9.0806) -> (121, 9.0806) construction
  circle A0 centre (83.1213, 6.9593) radius 1.35
  line L3 (9, 9.0806) -> (81, 9.0806) projected
  circle A1 centre (6.877, 6.9596) radius 1.35
  point P0 (4, 26.0806)
  dimension "d218" = 2.7
  dimension "d221" = 2.7
  constraints: 2 centre point, 2 end point, 1 horizontal
  measures "d218" diameter of A0
  measures "d221" diameter of A1
extrude "Extrusión43" cut sketch "Boceto59" against normal blind 43.5
sketch "Boceto60" plane through (42, 2.2425, 4) normal (0.750359, 0.6610305, 0) x (0, 0, -1)
  line L0 (81, 9.0806) -> (81, 34.0806) projected
  line L1 (81, 21.5806) -> (81, 15.5806)
  line L2 (81, 15.5806) -> (81, 27.5806)
  line L3 (84, 21.5806) -> (84, 20.0806)
  line L4 (84, 20.0806) -> (84, 23.0806)
  line L5 (84, 23.0806) -> (81, 27.5806)
  line L6 (84, 20.0806) -> (81, 15.5806)
  point P0 (4, 26.0806)
  dimension "d226" = 6
  dimension "d227" = 12
  dimension "d228" = 3
  dimension "d229" = 1.5
  dimension "d230" = 3
  constraints: 12 end point, 3 point on line, 1 midpoint
  measures "d226" distance of L1.start L1.end
  measures "d227" distance of L1.end L2.end
  measures "d228" distance of L1.start L3.start
  measures "d229" distance of L3.start L3.end
  measures "d230" distance of L3.end L4.end
extrude "Extrusión44" cut sketch "Boceto60" against normal blind 74
sketch "Boceto61" plane through (42, 2.2425, 4) normal (0.750359, 0.6610305, 0) x (0, 0, -1)
  line L0 (103, 15.0806) -> (103, 29)
  line L1 (103, 15.0806) -> (103, 15.5806)
  circle A0 centre (103, 15.5806) radius 1.35
  line L2 (103, 27.0806) -> (103, 30.0806)
  circle A1 centre (103, 30.0806) radius 1.35
  point P0 (4, 26.0806)
  point P1 (101, 15.0806)
  dimension "d233" = 2
  dimension "d234" = 0.5
  dimension "d235" = 2.7
  dimension "d236" = 3
  dimension "d237" = 2.7
  constraints: 6 end point, 3 point on line, 2 centre point, 2 coincident
  measures "d233" distance of point (101, 15.081) L0.start
  measures "d234" distance of L0.start L1.end
  measures "d235" diameter of A0
  measures "d236" distance of L2.start L2.end
  measures "d237" diameter of A1
extrude "Extrusión45" cut sketch "Boceto61" against normal blind 8.75
